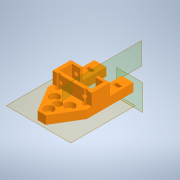
# Autodesk Inventor part: 30_Cube_Z_Focus_MGN12_NEMA_slide_part2_bolted
Saved by Autodesk Inventor 2022 (Build 260153000, 153)
## iProperties
Created: 2021-04-25
Part Number: 30_Cube_Z_Focus_MGN12_NEMA_slide_part2_bolted
Material: Generic
Document SubType Name: Modeling
Designer: diederichbenedict
Density: 1 g/cm^3
Appearance: Orange
Author: diederichbenedict
Autodesk Inventor part; units mm, degrees
ref_plane "YZ Plane" through (0, 0, 0) normal (1, 0, 0) x (0, 1, 0)
ref_plane "XZ Plane" through (0, 0, 0) normal (0, 1, 0) x (-1, 0, 0)
ref_plane "XY Plane" through (0, 0, 0) normal (0, 0, 1) x (1, 0, 0)
ref_plane "Work Plane8" through (-7.4556, -16.4352, 24.63) normal (0, 1, 0) x (0, 0, -1)
sketch "Sketch12" plane through (-7.4556, -16.4352, 24.63) normal (0, 1, 0) x (0, 0, -1)
  line L0 (59.1648, 4.9103) -> (72.1552, 12.4103) construction
  arc A0 (80.66, 7.5) -> (72.1552, 12.4103) centre (70.66, 0) ccw construction
  line L1 (80.66, 7.5) -> (80.66, -7.5) construction
  arc A1 (72.1552, -12.4103) -> (80.66, -7.5) centre (70.66, 0) ccw construction
  line L2 (72.1552, -12.4103) -> (59.1648, -4.9103) construction
  arc A2 (59.1648, 4.9103) -> (59.1648, -4.9103) centre (70.66, 0) ccw construction
  line L3 (57.3131, 5.945) -> (46.6951, 5.945) construction
  line L4 (46.6951, 5.945) -> (46.6951, -5.9961)
  line L5 (46.6951, -5.9961) -> (57.3131, -5.9961)
  line L6 (57.3131, -5.9961) -> (57.3131, -15)
  line L7 (57.3131, -15) -> (85.66, -15) construction
  line L8 (85.66, -15) -> (85.66, 15) construction
  line L9 (85.66, 15) -> (57.3131, 15) construction
  line L10 (57.3131, 15) -> (57.3131, 5.945) construction
  line L11 (46.6951, -6.3061) -> (57.3131, -6.3061)
  line L12 (41.63, -16.87) -> (45.71, -16.87) projected
  line L13 (55.66, -15) -> (46.2855, -13.3689) projected
  line L14 (55.66, -15) -> (105.1976, -15) construction
  line L15 (46.6951, 0) -> (46.6951, -6.3061)
  line L16 (9.71, -3.1754) -> (12.46, -1.5877) construction
  line L17 (12.46, -1.5877) -> (12.46, 1.5877) construction
  line L18 (12.46, 1.5877) -> (9.71, 3.1754) construction
  line L19 (9.71, 3.1754) -> (6.96, 1.5877) construction
  line L20 (6.96, 1.5877) -> (6.96, -1.5877) construction
  line L21 (6.96, -1.5877) -> (9.71, -3.1754) construction
  line L22 (-3.79, -3.4952) -> (-3.79, 3.4952)
  line L23 (-3.79, 0) -> (-3.79, 0)
  line L24 (-3.79, 0) -> (-3.79, -3.4952)
  line L25 (-3.79, -3.4952) -> (17.9117, -16.5162)
  line L26 (46.6951, 0) -> (-3.79, 0)
  line L27 (57.3131, -6.3061) -> (57.3131, -15)
  line L28 (57.3131, -15) -> (37.3669, -15)
  line L29 (-3.79, -8.16) -> (-3.79, 8.16) projected
  line L30 (19.46, 16.4952) -> (10.1021, 16.4952) projected
  line L31 (19.46, -16.4952) -> (19.46, 16.4952) projected
  line L32 (10.1021, -16.4952) -> (19.46, -16.4952) projected
  line L33 (10.1021, 16.4952) -> (-3.79, 8.16) projected
  line L34 (-3.79, -8.16) -> (10.1021, -16.4952) projected
  line L35 (17.9117, -16.5162) -> (57.3131, -16.5162)
  line L36 (57.3131, -16.5162) -> (57.3131, -15)
  line L37 (57.3131, -15) -> (37.3669, -15)
  line L38 (39.63, 0) -> (49.93, 0)
  line L39 (49.93, 0) -> (49.93, -12.8511)
  line L40 (49.93, -12.8511) -> (39.63, -12.8511)
  line L41 (39.63, -12.8511) -> (39.63, 0)
  line L42 (52.63, -16.0211) -> (18.69, -16.0211) construction
  line L43 (18.69, 17.9189) -> (52.63, 17.9189) projected
  arc A3 (48.3173, -4.8992) -> (48.4594, -5.1011) centre (48.5983, -4.8523) ccw projected
  line L44 (48.4594, -5.1011) -> (52.63, -5.1011) projected
  line L45 (52.63, -5.1011) -> (52.63, 6.9989) projected
  line L46 (48.4594, 6.9989) -> (52.63, 6.9989) projected
  arc A4 (48.4594, 6.9989) -> (48.3173, 6.7971) centre (48.5983, 6.7502) ccw projected
  arc A5 (47.9241, 6.5003) -> (48.3173, 6.7971) centre (47.4153, 7.5832) ccw projected
  arc A6 (47.9241, 6.5003) -> (47.8129, 6.374) centre (48.0446, 6.2821) ccw projected
  line L47 (47.7741, 5.8769) -> (47.8129, 6.374) projected
  arc A7 (47.5555, 5.6489) -> (47.7741, 5.8769) centre (47.5256, 5.8964) ccw projected
  line L48 (47.1044, 5.6489) -> (47.5555, 5.6489) projected
  arc A8 (46.8561, 5.8765) -> (47.1044, 5.6489) centre (47.1044, 5.8982) ccw projected
  line L49 (46.8241, 6.242) -> (46.8561, 5.8765) projected
  arc A9 (46.8241, 6.242) -> (46.6712, 6.5003) centre (46.5764, 6.2698) ccw projected
  arc A10 (46.1533, 6.8443) -> (46.6712, 6.5003) centre (47.0626, 7.6514) ccw projected
  arc A11 (46.1533, 6.8443) -> (45.93, 6.9989) centre (45.9227, 6.7498) ccw projected
  line L50 (45.33, 6.9989) -> (45.93, 6.9989) projected
  line L51 (44.83, 6.4989) -> (45.33, 6.9989) projected
  line L52 (44.83, 6.4989) -> (44.83, -4.6011) projected
  line L53 (44.83, -4.6011) -> (45.33, -5.1011) projected
  line L54 (45.33, -5.1011) -> (45.93, -5.1011) projected
  arc A12 (45.93, -5.1011) -> (46.1533, -4.9464) centre (45.9227, -4.8519) ccw projected
  arc A13 (46.6712, -4.6024) -> (46.1533, -4.9464) centre (47.0626, -5.7535) ccw projected
  arc A14 (46.6712, -4.6024) -> (46.8241, -4.3441) centre (46.5764, -4.3719) ccw projected
  line L55 (46.8241, -4.3441) -> (46.8561, -3.9786) projected
  arc A15 (47.1044, -3.7511) -> (46.8561, -3.9786) centre (47.1044, -4.0003) ccw projected
  line L56 (47.1044, -3.7511) -> (47.5555, -3.7511) projected
  arc A16 (47.7741, -3.9791) -> (47.5555, -3.7511) centre (47.5256, -3.9985) ccw projected
  line L57 (47.7741, -3.9791) -> (47.8129, -4.4761) projected
  arc A17 (47.8129, -4.4761) -> (47.9241, -4.6024) centre (48.0446, -4.3842) ccw projected
  arc A18 (48.3173, -4.8992) -> (47.9241, -4.6024) centre (47.4153, -5.6854) ccw projected
  arc A19 (48.2566, -4.8959) -> (47.7572, -4.3183) centre (47.1462, -5.3511) ccw construction
  arc A20 (47.6355, -4.1249) -> (47.7572, -4.3183) centre (47.8845, -4.1031) ccw construction
  line L58 (47.6355, -4.1249) -> (47.6053, -3.7793) construction
  arc A21 (47.6053, -3.7793) -> (47.3562, -3.5511) centre (47.3562, -3.8011) ccw construction
  line L59 (47.3562, -3.5511) -> (46.9038, -3.5511) construction
  arc A22 (46.9038, -3.5511) -> (46.6547, -3.7793) centre (46.9038, -3.8011) ccw construction
  line L60 (46.6547, -3.7793) -> (46.6227, -4.1458) construction
  arc A23 (46.5068, -4.3356) -> (46.6227, -4.1458) centre (46.3736, -4.124) ccw construction
  arc A24 (46.5068, -4.3356) -> (46.0359, -4.8959) centre (47.1462, -5.3511) ccw construction
  arc A25 (45.8046, -5.0511) -> (46.0359, -4.8959) centre (45.8046, -4.8011) ccw construction
  line L61 (45.8046, -5.0511) -> (45.13, -5.0511) construction
  line L62 (45.13, -5.0511) -> (44.63, -4.5511) construction
  line L63 (44.63, -4.5511) -> (44.63, 6.4489) construction
  line L64 (44.63, 6.4489) -> (45.13, 6.9489) construction
  line L65 (45.13, 6.9489) -> (45.8046, 6.9489) construction
  arc A26 (46.0359, 6.7938) -> (45.8046, 6.9489) centre (45.8046, 6.6989) ccw construction
  arc A27 (46.0359, 6.7938) -> (46.5068, 6.2335) centre (47.1462, 7.2489) ccw construction
  arc A28 (46.6227, 6.0437) -> (46.5068, 6.2335) centre (46.3736, 6.0219) ccw construction
  line L66 (46.6227, 6.0437) -> (46.6547, 5.6771) construction
  arc A29 (46.6547, 5.6771) -> (46.9038, 5.4489) centre (46.9038, 5.6989) ccw construction
  line L67 (46.9038, 5.4489) -> (47.3562, 5.4489) construction
  arc A30 (47.3562, 5.4489) -> (47.6053, 5.6771) centre (47.3562, 5.6989) ccw construction
  line L68 (47.6053, 5.6771) -> (47.6355, 6.0228) construction
  arc A31 (47.7572, 6.2161) -> (47.6355, 6.0228) centre (47.8845, 6.001) ccw construction
  arc A32 (47.7572, 6.2161) -> (48.2566, 6.7938) centre (47.1462, 7.2489) ccw construction
  arc A33 (48.4879, 6.9489) -> (48.2566, 6.7938) centre (48.4879, 6.6989) ccw construction
  line L69 (48.4879, 6.9489) -> (49.63, 6.9489) construction
  line L70 (49.63, 6.9489) -> (49.63, 13.8489) construction
  line L71 (49.63, 13.8489) -> (49.03, 14.4489) construction
  line L72 (49.03, 14.4489) -> (45.63, 14.4489) construction
  arc A34 (44.83, 14.4489) -> (45.63, 14.4489) centre (45.23, 14.7489) ccw construction
  line L73 (44.83, 14.4489) -> (40.23, 14.4489) construction
  line L74 (40.23, 14.4489) -> (39.63, 13.8489) construction
  line L75 (39.63, 13.8489) -> (39.63, 7.3489) construction
  line L76 (39.63, 7.3489) -> (40.03, 6.9489) construction
  line L77 (40.03, 6.9489) -> (40.03, -5.0511) construction
  line L78 (40.03, -5.0511) -> (39.63, -5.4511) construction
  line L79 (39.63, -5.4511) -> (39.63, -11.951) construction
  line L80 (39.63, -11.951) -> (40.23, -12.5511) construction
  line L81 (40.23, -12.5511) -> (49.03, -12.5511) construction
  line L82 (49.03, -12.5511) -> (49.63, -11.9511) construction
  line L83 (49.63, -11.9511) -> (49.63, -5.0511) construction
  line L84 (49.63, -5.0511) -> (48.4879, -5.0511) construction
  arc A35 (48.2566, -4.8959) -> (48.4879, -5.0511) centre (48.4879, -4.8011) ccw construction
  point P0 (24.63, -7.4556)
  point P1 (11.21, -12.4952)
  point P2 (19.46, 12.4952)
  point P3 (19.46, -12.4952)
  dimension "d114" = 5.1011
  dimension "d115" = 6.9989
  dimension "d116" = 0.3
  dimension "d117" = 0.3
  constraints: 40 end point, 7 point on line, 3 horizontal, 3 parallel, 3 perpendicular, 3 vertical, 1 coincident, 1 collinear, 1 midpoint, 2 other
  measures "d114" distance between parallel lines of L26 L44
  measures "d115" distance between parallel lines of L46 L26
  measures "d116" distance between parallel lines of L81 L40
  measures "d117" distance from line of L82.end L39
extrude "Extrusion11" add sketch "Sketch12" along normal blind 7 contours L38 L39 L44 A3 A18 A17 L57 A16 L56 A15 L55 A14 L4 | L4 A14 A13 A12 L54 L53 L52 L26 | A14 L55 A15 L56 A16 L57 A17 A18 A3 L44 L39 L5 L4 | L4 L15 L11 L39 L40 L41 L26 L52 L53 L54 A12 A13 A14 | L5 L39 L11 L15 | L41 L40 L39 L11 L6 L36 L35 L25 L32 L31 L26 | L31 L32 L25 L22 L26
sketch "Sketch13" plane through (-7.4556, -9.4352, 24.63) normal (0, 1, 0) x (1, 0, 0)
  line L0 (-13.1744, 24.9113) -> (13.5, 24.9113)
  line L1 (13.5, 24.9113) -> (13.5, 35.2113)
  line L2 (13.5, 35.2113) -> (-13.1744, 35.2113)
  line L3 (-13.1744, 35.2113) -> (-13.1744, 24.9113)
  line L4 (-13.5, 34.3113) -> (-13.5, 26.5113) construction
  line L5 (-13.5, 26.5113) -> (-12.3, 25.3113) construction
  line L6 (-12.3, 25.3113) -> (11.7, 25.3113) construction
  line L7 (11.7, 25.3113) -> (12.9, 26.5113) construction
  line L8 (12.9, 26.5113) -> (12.9, 34.3113) construction
  line L9 (12.9, 34.3113) -> (12.3, 34.9113) construction
  line L10 (12.3, 34.9113) -> (5.7, 34.9113) construction
  line L11 (5.7, 34.9113) -> (5.7, 33.7692) construction
  arc A0 (5.5448, 33.5379) -> (5.7, 33.7692) centre (5.45, 33.7692) ccw construction
  arc A1 (5.5448, 33.5379) -> (4.9672, 33.0386) centre (6, 32.4276) ccw construction
  arc A2 (4.7738, 32.9168) -> (4.9672, 33.0386) centre (4.752, 33.1659) ccw construction
  line L12 (4.7738, 32.9168) -> (4.4282, 32.8866) construction
  arc A3 (4.4282, 32.8866) -> (4.2, 32.6375) centre (4.45, 32.6375) ccw construction
  line L13 (4.2, 32.6375) -> (4.2, 32.1851) construction
  arc A4 (4.2, 32.1851) -> (4.4282, 31.9361) centre (4.45, 32.1851) ccw construction
  line L14 (4.4282, 31.9361) -> (4.7947, 31.904) construction
  arc A5 (4.9845, 31.7882) -> (4.7947, 31.904) centre (4.773, 31.6549) ccw construction
  arc A6 (4.9845, 31.7882) -> (5.5448, 31.3172) centre (6, 32.4276) ccw construction
  arc A7 (5.7, 31.0859) -> (5.5448, 31.3172) centre (5.45, 31.0859) ccw construction
  line L15 (5.7, 31.0859) -> (5.7, 30.4113) construction
  line L16 (5.7, 30.4113) -> (5.2, 29.9113) construction
  line L17 (5.2, 29.9113) -> (-5.8, 29.9113) construction
  line L18 (-5.8, 29.9113) -> (-6.3, 30.4113) construction
  line L19 (-6.3, 30.4113) -> (-6.3, 31.0859) construction
  arc A8 (-6.1448, 31.3172) -> (-6.3, 31.0859) centre (-6.05, 31.0859) ccw construction
  arc A9 (-6.1448, 31.3172) -> (-5.5845, 31.7882) centre (-6.6, 32.4276) ccw construction
  arc A10 (-5.3948, 31.904) -> (-5.5845, 31.7882) centre (-5.373, 31.6549) ccw construction
  line L20 (-5.3948, 31.904) -> (-5.0282, 31.9361) construction
  arc A11 (-5.0282, 31.9361) -> (-4.8, 32.1851) centre (-5.05, 32.1851) ccw construction
  line L21 (-4.8, 32.1851) -> (-4.8, 32.6375) construction
  arc A12 (-4.8, 32.6375) -> (-5.0282, 32.8866) centre (-5.05, 32.6375) ccw construction
  line L22 (-5.0282, 32.8866) -> (-5.3738, 32.9168) construction
  arc A13 (-5.5672, 33.0386) -> (-5.3738, 32.9168) centre (-5.352, 33.1659) ccw construction
  arc A14 (-5.5672, 33.0386) -> (-6.1448, 33.5379) centre (-6.6, 32.4276) ccw construction
  arc A15 (-6.3, 33.7692) -> (-6.1448, 33.5379) centre (-6.05, 33.7692) ccw construction
  line L23 (-6.3, 33.7692) -> (-6.3, 34.9113) construction
  line L24 (-6.3, 34.9113) -> (-12.9, 34.9113) construction
  line L25 (-12.9, 34.9113) -> (-13.5, 34.3113) construction
  circle A16 centre (-7.2, 27.9063) radius 2.1 construction
  circle A17 centre (6.6, 27.9063) radius 2.1 construction
  arc A18 (5.5448, 33.5379) -> (4.9672, 33.0386) centre (6, 32.4276) ccw construction
  arc A19 (4.7738, 32.9168) -> (4.9672, 33.0386) centre (4.752, 33.1659) ccw construction
  line L26 (4.7738, 32.9168) -> (4.4282, 32.8866) construction
  arc A20 (4.4282, 32.8866) -> (4.2, 32.6375) centre (4.45, 32.6375) ccw construction
  line L27 (4.2, 32.6375) -> (4.2, 32.1851) construction
  arc A21 (4.2, 32.1851) -> (4.4282, 31.9361) centre (4.45, 32.1851) ccw construction
  line L28 (4.4282, 31.9361) -> (4.7948, 31.904) construction
  arc A22 (4.9845, 31.7882) -> (4.7948, 31.904) centre (4.773, 31.6549) ccw construction
  arc A23 (4.9845, 31.7882) -> (5.5448, 31.3172) centre (6, 32.4276) ccw construction
  arc A24 (5.7, 31.0859) -> (5.5448, 31.3172) centre (5.45, 31.0859) ccw construction
  line L29 (5.7, 31.0859) -> (5.7, 30.4113) construction
  line L30 (5.7, 30.4113) -> (5.2, 29.9113) construction
  line L31 (5.2, 29.9113) -> (-5.8, 29.9113) construction
  line L32 (-5.8, 29.9113) -> (-6.3, 30.4113) construction
  line L33 (-6.3, 30.4113) -> (-6.3, 31.0859) construction
  arc A25 (-6.1448, 31.3172) -> (-6.3, 31.0859) centre (-6.05, 31.0859) ccw construction
  arc A26 (-6.1448, 31.3172) -> (-5.5846, 31.7882) centre (-6.6, 32.4276) ccw construction
  arc A27 (-5.3948, 31.904) -> (-5.5846, 31.7882) centre (-5.373, 31.6549) ccw construction
  line L34 (-5.3948, 31.904) -> (-5.0282, 31.9361) construction
  arc A28 (-5.0282, 31.9361) -> (-4.8, 32.1851) centre (-5.05, 32.1851) ccw construction
  line L35 (-4.8, 32.1851) -> (-4.8, 32.6375) construction
  arc A29 (-4.8, 32.6375) -> (-5.0282, 32.8866) centre (-5.05, 32.6375) ccw construction
  line L36 (-5.0282, 32.8866) -> (-5.3738, 32.9168) construction
  arc A30 (-5.5672, 33.0386) -> (-5.3738, 32.9168) centre (-5.3521, 33.1659) ccw construction
  arc A31 (-5.5672, 33.0386) -> (-6.1448, 33.5379) centre (-6.6, 32.4276) ccw construction
  arc A32 (-6.3, 33.7692) -> (-6.1448, 33.5379) centre (-6.05, 33.7692) ccw construction
  line L37 (-6.3, 33.7692) -> (-6.3, 34.9113) construction
  line L38 (-6.3, 34.9113) -> (-13.2, 34.9113) construction
  line L39 (-13.2, 34.9113) -> (-13.8, 34.3113) construction
  line L40 (-13.8, 34.3113) -> (-13.8, 30.9113) construction
  arc A33 (-13.8, 30.1113) -> (-13.8, 30.9113) centre (-14.1, 30.5113) ccw construction
  line L41 (-13.8, 30.1113) -> (-13.8, 25.5113) construction
  line L42 (-13.8, 25.5113) -> (-13.2, 24.9113) construction
  line L43 (-13.2, 24.9113) -> (-6.7, 24.9113) construction
  line L44 (-6.7, 24.9113) -> (-6.3, 25.3113) construction
  line L45 (-6.3, 25.3113) -> (5.7, 25.3113) construction
  line L46 (5.7, 25.3113) -> (6.1, 24.9113) construction
  line L47 (6.1, 24.9113) -> (12.6, 24.9113) construction
  line L48 (12.6, 24.9113) -> (13.2, 25.5113) construction
  line L49 (13.2, 25.5113) -> (13.2, 34.3113) construction
  line L50 (13.2, 34.3113) -> (12.6, 34.9113) construction
  line L51 (12.6, 34.9113) -> (5.7, 34.9113) construction
  line L52 (5.7, 34.9113) -> (5.7, 33.7692) construction
  arc A34 (5.5448, 33.5379) -> (5.7, 33.7692) centre (5.45, 33.7692) ccw construction
  point P0 (7.4556, 24.63)
  dimension "d110" = 0.3
  dimension "d111" = 0.3
  constraints: 8 end point, 2 parallel, 1 horizontal, 1 perpendicular, 1 point on line
  measures "d110" distance between parallel lines of L49 L1
  measures "d111" distance between parallel lines of L2 L10
extrude "Extrusion12" cut sketch "Sketch13" against normal through all
mirror "Mirror3" about plane through (-7.4556, -16.4352, -22.0651) normal (-1, 0, 0) of "Extrusion11", "Extrusion12"
sketch "Sketch17" plane through (-7.4556, -9.4352, 24.63) normal (0, 1, 0) x (1, 0, 0)
  circle A0 centre (6.4952, 13.46) radius 4 projected
  circle A1 centre (0, 2.21) radius 4 projected
  circle A2 centre (-6.4952, 13.46) radius 4 projected
  point P0 (7.4556, 24.63)
extrude "Extrusion16" cut sketch "Sketch17" against normal blind 4.5
sketch "Sketch18" plane through (-7.4556, -9.4352, 24.63) normal (0, 1, 0) x (1, 0, 0)
  line L0 (-16.5162, 17.9117) -> (-16.5162, 57.3131) projected
  line L1 (16.5162, 17.9117) -> (16.5162, 57.3131) projected
  line L2 (16.5162, 26.0101) -> (16.5162, 22.0101)
  line L3 (16.5162, 22.0101) -> (-16.5162, 22.0101)
  line L4 (-16.5162, 22.0101) -> (-16.5162, 26.0101)
  line L5 (15, 57.3131) -> (15, 37.2259) projected
  line L6 (-15, 37.2259) -> (15, 37.2259) construction
  line L7 (-16.5162, 37.361) -> (16.5162, 37.361)
  line L8 (16.5162, 17.9117) -> (16.5162, 57.3131) projected
  line L9 (-16.5162, 37.361) -> (16.5162, 37.361) construction
  line L10 (-13.5, 35.2113) -> (13.5, 35.2113)
  line L11 (13.5, 35.2113) -> (13.5, 24.9113)
  line L12 (13.5, 24.9113) -> (-13.5, 24.9113)
  line L13 (-13.5, 24.9113) -> (-13.5, 35.2113)
  line L14 (-16.5162, 37.361) -> (16.5162, 37.361)
  line L15 (16.5162, 37.361) -> (16.5162, 22.0101)
  line L16 (16.5162, 22.0101) -> (-16.5162, 22.0101)
  line L17 (-16.5162, 22.0101) -> (-16.5162, 37.361)
  point P0 (7.4556, 24.63)
  point P1 (15, 37.3669)
  dimension "d85" = 4
  dimension "d96" = 0
  constraints: 28 end point, 5 parallel, 4 horizontal, 4 point on line, 2 perpendicular, 1 collinear
  measures "d85" distance of L2.start L2.end
  measures "d96" distance between parallel lines of L7 L9
extrude "Extrusion17" add sketch "Sketch18" along normal blind 10
sketch "Sketch20" plane through (-7.4556, -9.4352, 24.63) normal (0, 1, 0) x (1, 0, 0)
  circle A0 centre (-10.5315, 68.5467) radius 1.4 projected
  circle A1 centre (8.7824, 68.5467) radius 1.4 projected
  arc A2 (-10.1298, 62.2055) -> (-10.9331, 62.2055) centre (-10.5315, 63.5467) ccw projected
  arc A3 (9.1841, 62.2055) -> (8.3808, 62.2055) centre (8.7824, 63.5467) ccw projected
  circle A4 centre (-10.5315, 63.5467) radius 1.4
  circle A5 centre (8.7824, 63.5467) radius 1.4
  point P0 (7.4556, 24.63)
  constraints: 2 centre point, 2 coincident, 2 concentric
extrude "Extrusion18" cut sketch "Sketch20" against normal blind 10
sketch "Sketch21" plane through (-7.4556, 0.5648, 24.63) normal (0, 1, 0) x (1, 0, 0)
  line L0 (-13.1744, 33.91) -> (-13.1744, 26.11) projected
  line L1 (-13.1744, 26.11) -> (-11.9744, 24.91) projected
  line L2 (-11.9744, 24.91) -> (12.0256, 24.91) projected
  line L3 (12.0256, 24.91) -> (13.2256, 26.11) projected
  line L4 (13.2256, 26.11) -> (13.2256, 33.91) projected
  line L5 (13.2256, 33.91) -> (12.6256, 34.51) projected
  line L6 (12.6256, 34.51) -> (6.0256, 34.51) projected
  line L7 (6.0256, 34.51) -> (6.0256, 33.3679) projected
  arc A0 (5.8704, 33.1366) -> (6.0256, 33.3679) centre (5.7756, 33.3679) ccw projected
  arc A1 (5.8704, 33.1366) -> (5.2928, 32.6373) centre (6.3256, 32.0262) ccw projected
  arc A2 (5.0994, 32.5155) -> (5.2928, 32.6373) centre (5.0776, 32.7645) ccw projected
  line L8 (5.0994, 32.5155) -> (4.7538, 32.4853) projected
  arc A3 (4.7538, 32.4853) -> (4.5256, 32.2362) centre (4.7756, 32.2362) ccw projected
  line L9 (4.5256, 32.2362) -> (4.5256, 31.7838) projected
  arc A4 (4.5256, 31.7838) -> (4.7538, 31.5348) centre (4.7756, 31.7838) ccw projected
  line L10 (4.7538, 31.5348) -> (5.1203, 31.5027) projected
  arc A5 (5.3101, 31.3868) -> (5.1203, 31.5027) centre (5.0985, 31.2536) ccw projected
  arc A6 (5.3101, 31.3868) -> (5.8704, 30.9159) centre (6.3256, 32.0262) ccw projected
  arc A7 (6.0256, 30.6846) -> (5.8704, 30.9159) centre (5.7756, 30.6846) ccw projected
  line L11 (6.0256, 30.6846) -> (6.0256, 30.01) projected
  line L12 (6.0256, 30.01) -> (5.5256, 29.51) projected
  line L13 (5.5256, 29.51) -> (-5.4744, 29.51) projected
  line L14 (-5.4744, 29.51) -> (-5.9744, 30.01) projected
  line L15 (-5.9744, 30.01) -> (-5.9744, 30.6846) projected
  arc A8 (-5.8192, 30.9159) -> (-5.9744, 30.6846) centre (-5.7244, 30.6846) ccw projected
  arc A9 (-5.8192, 30.9159) -> (-5.259, 31.3868) centre (-6.2744, 32.0262) ccw projected
  arc A10 (-5.0692, 31.5027) -> (-5.259, 31.3868) centre (-5.0474, 31.2536) ccw projected
  line L16 (-5.0692, 31.5027) -> (-4.7026, 31.5347) projected
  arc A11 (-4.7026, 31.5347) -> (-4.4744, 31.7838) centre (-4.7244, 31.7838) ccw projected
  line L17 (-4.4744, 31.7838) -> (-4.4744, 32.2362) projected
  arc A12 (-4.4744, 32.2362) -> (-4.7026, 32.4853) centre (-4.7244, 32.2362) ccw projected
  line L18 (-4.7026, 32.4853) -> (-5.0482, 32.5155) projected
  arc A13 (-5.2416, 32.6373) -> (-5.0482, 32.5155) centre (-5.0265, 32.7645) ccw projected
  arc A14 (-5.2416, 32.6373) -> (-5.8192, 33.1366) centre (-6.2744, 32.0262) ccw projected
  arc A15 (-5.9744, 33.3679) -> (-5.8192, 33.1366) centre (-5.7244, 33.3679) ccw projected
  line L19 (-5.9744, 33.3679) -> (-5.9744, 34.51) projected
  line L20 (-5.9744, 34.51) -> (-12.5744, 34.51) projected
  line L21 (-12.5744, 34.51) -> (-13.1744, 33.91) projected
  circle A16 centre (-6.8744, 27.505) radius 2.1 projected
  circle A17 centre (6.9256, 27.505) radius 2.1 projected
  line L22 (-6.4744, 28.46) -> (6.5256, 28.46)
  line L23 (6.5256, 28.46) -> (6.5256, 59.0305)
  line L24 (6.5256, 59.0305) -> (-6.4744, 59.0305)
  line L25 (-6.4744, 59.0305) -> (-6.4744, 28.46)
  point P0 (7.4556, 24.63)
  dimension "d99" = 0.5
  dimension "d100" = 0.5
  constraints: 8 end point, 2 parallel, 1 horizontal, 1 perpendicular
  measures "d99" distance between parallel lines of L19 L25
  measures "d100" distance from line of L23 L6.end
extrude "Extrusion19" cut sketch "Sketch21" against normal through all contours L25 L24 L23 L6 L7 A0 A1 A2 L8 A3 L9 A4 L10 A5 A6 A7 L11 L12 L13 L14 L15 A8 A9 A10 L16 A11 L17 A12 L18 A13 A14 A15 L19 L20 | L20 L19 A15 A14 A13 L18 A12 L17 A11 L16 A10 A9 A8 L15 L14 L13 L12 L11 A7 A6 A5 L10 A4 L9 A3 L8 A2 A1 A0 L7 L6 L23 A17 L22 A16 L25 | A16 L22 L25 | A17 L23 L22 picked at (-5.5817, 28.592) picked at (5.6329, 28.592)
sketch "Sketch22" plane through (-7.4556, -9.4352, 24.63) normal (0, 1, 0) x (1, 0, 0)
  circle A0 centre (-0.9489, 24.63) radius 3
  circle A1 centre (-0.9489, 24.63) radius 1.5 projected
  point P0 (7.4556, 24.63)
  dimension "d103" = 6
  constraints: 1 centre point
  measures "d103" diameter of A0
extrude "Extrusion20" cut sketch "Sketch22" against normal blind 10 contours A0 | A1
sketch "Sketch23" plane through (-7.4556, -9.4352, 24.63) normal (0, 1, 0) x (1, 0, 0)
  circle A0 centre (11.5, 21.21) radius 1.025 projected
  circle A1 centre (-11.5, 21.21) radius 1.25 projected
  circle A2 centre (11.5, 21.21) radius 1.75
  circle A3 centre (-11.5, 21.21) radius 1.75
  point P0 (7.4556, 24.63)
  dimension "d106" = 3.5
  dimension "d107" = 3.5
  constraints: 2 centre point, 2 coincident
  measures "d106" diameter of A2
  measures "d107" diameter of A3
extrude "Extrusion21" cut sketch "Sketch23" along normal through all both and the other way through all contours A0 | A1 | A2 | A3
ref_plane "Arbeitsebene9" through (5.8531, -16.4352, -32.6831) normal (0, 0, -1) x (-1, 0, 0)
sketch "Skizze24" plane through (5.8531, -16.4352, -32.6831) normal (0, 0, -1) x (-1, 0, 0)
  line L0 (6.7831, 0) -> (6.7831, 7) projected
  line L1 (-3.2076, 7) -> (6.7831, 7) projected
  line L2 (-3.2076, 0) -> (6.7831, 0) projected
  line L3 (19.7831, 7) -> (19.7831, 0) projected
  line L4 (29.8249, 0) -> (19.7831, 0) projected
  line L5 (29.8249, 7) -> (19.7831, 7) projected
  circle A0 centre (24.8086, 3.5) radius 1.4
  circle A1 centre (1.8086, 3.5) radius 1.4
  circle A2 centre (1.8086, 3.5) radius 3.5
  circle A3 centre (24.8086, 3.5) radius 3.5
  line L6 (29.8249, 0) -> (29.8249, 7) projected
  line L7 (-3.2076, 0) -> (-3.2076, 7) projected
  point P0 (5.8531, 16.4352)
  dimension "d118" = 2.8
  dimension "d119" = 2.8
  constraints: 4 centre point, 4 tangent, 2 coincident
  measures "d118" diameter of A0
  measures "d119" diameter of A1
extrude "Extrusion22" cut sketch "Skizze24" against normal up to surface (32.4018 mm away) contours A0 | A1
sketch "Skizze25" plane through (-7.4556, -9.4352, 24.63) normal (0, 1, 0) x (1, 0, 0)
  point P0 (7.4556, 24.63)
ref_plane "Work Plane10" through (-7.4556, -16.4352, -32.6831) normal (-1, 0, 0) x (0, 0, 1)
sketch "Sketch26" plane through (-7.4556, -9.4352, 24.63) normal (0, 1, 0) x (1, 0, 0)
  line L0 (12.9, 57.3131) -> (12.9, 35.2113) projected
  line L1 (10.1, 57.3131) -> (10.1, 35.2113) projected
  line L2 (-10.1, 57.3131) -> (-10.1, 35.2113) projected
  line L3 (-12.9, 57.3131) -> (-12.9, 35.2113) projected
  line L4 (8.75, 46.9665) -> (14.25, 46.9665)
  line L5 (14.25, 46.9665) -> (14.25, 49.9665)
  line L6 (14.25, 49.9665) -> (8.75, 49.9665)
  line L7 (8.75, 49.9665) -> (8.75, 46.9665)
  line L8 (8.75, 46.9665) -> (14.25, 49.9665) construction
  line L9 (14.25, 46.9665) -> (8.75, 49.9665) construction
  line L10 (-14.25, 46.9665) -> (-8.75, 46.9665)
  line L11 (-8.75, 46.9665) -> (-8.75, 49.9665)
  line L12 (-8.75, 49.9665) -> (-14.25, 49.9665)
  line L13 (-14.25, 49.9665) -> (-14.25, 46.9665)
  line L14 (-14.25, 46.9665) -> (-8.75, 49.9665) construction
  line L15 (-8.75, 46.9665) -> (-14.25, 49.9665) construction
  point P0 (7.4556, 24.63)
  point P1 (11.5, 48.4665)
  point P2 (-11.5, 48.4665)
  dimension "d122" = 5.5
  dimension "d123" = 3
  dimension "d124" = 5.5
  dimension "d125" = 1.4
  dimension "d126" = 1.4
  dimension "d127" = 2.8
  constraints: 24 end point, 4 midpoint, 4 parallel, 2 horizontal, 2 perpendicular, 1 point on line
  measures "d122" distance of L6.end L5.end
  measures "d123" distance of L5.end L4.end
  measures "d124" distance of L12.end L11.end
  measures "d125" distance from line of point (-11.5, 48.467) L3
  measures "d126" distance from line of L1 point (11.5, 48.467)
  measures "d127" distance between parallel lines of L1 L0
extrude "Extrusion23" cut sketch "Sketch26" against normal blind 10
sketch "Sketch27" plane through (-9.8661, -9.4352, 2.6199) normal (0, 0, 1) x (1, 0, 0)
  line L0 (15.6605, -7) -> (12.1605, -7) projected
  circle A0 centre (-7.5895, 4.3) radius 1.5 projected
  circle A1 centre (12.4105, 4.3) radius 1.75 projected
  point P0 (9.8661, 9.4352)
hole "Hole2" at (-17.4556, -5.1352, 2.6199) at (2.5444, -5.1352, 2.6199) direction (0, 0, -1) diameter 3 end through all
sketch "Skizze28" plane through (-7.4556, -9.4352, 24.63) normal (0, 1, 0) x (1, 0, 0)
  circle A0 centre (6.4952, 13.46) radius 4 projected
  circle A1 centre (-6.4952, 13.46) radius 4 projected
  circle A2 centre (0, 2.21) radius 4 projected
  line L0 (6.4952, 13.46) -> (0, 2.21) construction
  line L1 (0, 2.21) -> (-6.4952, 13.46) construction
  line L2 (-6.4952, 13.46) -> (6.4952, 13.46) construction
  circle A3 centre (0, 9.71) radius 3.75 construction
  circle A4 centre (0, 9.71) radius 3.2023
  point P0 (7.4556, 24.63)
  constraints: 6 end point, 3 tangent, 2 centre point, 1 horizontal
extrude "Extrusion24" cut sketch "Skizze28" against normal blind 10 contours A4
equation "\"d124\" = d122"
equation "\"d125\" = 0.5 * d127"
equation "\"d126\" = 0.5 * d127"
body "Solid2"
